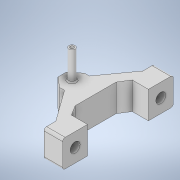
# Autodesk Inventor part: Base 2 LMU8
Saved by Autodesk Inventor 2022 (Build 260153000, 153)
## iProperties
Created: 2022-02-16
Part Number: Base 2 LMU8
Material: Genérico
Document SubType Name: Modeling
Designer: mathe
Density: 1 g/cm^3
Appearance: Padrão
Author: mathe
## iProperties of the stored document Base 2 LMU8_3DPrint.ipt
Created: 2022-02-18
Part Number: Base 2 LMU8_3DPrint
Material: Genérico
Document SubType Name: Modeling
Designer: mathe
Density: 1 g/cm^3
Appearance: Padrão
Author: mathe
Autodesk Inventor part; units mm, degrees
ref_plane "YZ Plane" through (0, 0, 0) normal (1, 0, 0) x (0, 1, 0)
ref_plane "XZ Plane" through (0, 0, 0) normal (0, 1, 0) x (-1, 0, 0)
ref_plane "XY Plane" through (0, 0, 0) normal (0, 0, 1) x (1, 0, 0)
sketch "Esboço1" plane through (0, 0, 0) normal (0, 1, 0) x (-1, 0, 0)
  line L0 (0, 0) -> (22, 0)
  line L1 (22, 0) -> (22, -22)
  line L2 (22, -22) -> (0, -22)
  line L3 (0, -22) -> (0, 0)
  dimension "d0" = 22
  dimension "d1" = 22
  constraints: 8 end point, 2 parallel, 1 horizontal, 1 perpendicular
  measures "d0" distance of L1.end L2.end
  measures "d1" distance of L0.end L1.end
extrude "Extrusão1" add sketch "Esboço1" along normal blind 20
sketch "Esboço2" plane through (0, 20, 0) normal (0, 1, 0) x (1, 0, 0)
  point P0 (0, 0)
  point P1 (-11, 11)
hole "Furo1" at (-11, 20, -11) direction (0, -1, 0) diameter 15 end through all
sketch "Esboço3" plane through (-22, 0, -22) normal (-1, 0, 0) x (0, 0, 1)
  line L0 (22, 0) -> (22, 20) projected
  line L1 (22, 10) -> (22, -34.5)
  line L2 (22, 10) -> (22, 54.5)
  line L3 (22, -34.5) -> (37, -34.5)
  line L4 (37, -34.5) -> (37, 54.5)
  line L5 (37, 54.5) -> (22, 54.5)
  line L6 (22, 54.5) -> (22, -34.5)
  dimension "d13" = 15
  constraints: 12 end point, 2 parallel, 1 collinear, 1 horizontal, 1 midpoint, 1 perpendicular, 1 point on line
  measures "d13" distance of L5.end L4.end
extrude "Extrusão2" add sketch "Esboço3" against normal up to surface (22 mm away)
chamfer "Chanfro1" distance 18 distance2 25 1 edges at (-11, 0, 0) measured on face at (-11, 0, -0.5)
sketch "Esboço4" plane through (-22, -34.5, 15) normal (0, 0, 1) x (1, 0, 0)
  line L0 (0, 89) -> (22, 89) projected
  point P0 (22, 34.5)
  point P1 (11, 10)
  point P2 (11, 79)
  dimension "d20" = 10
  measures "d20" distance from line of L0 point (11, 79)
hole "Furo2" at (-11, -24.5, 15) at (-11, 44.5, 15) direction (0, 0, -1) diameter 8 end through all
chamfer "Chanfro3" distance 18 distance2 25 1 edges at (-11, 20, 0) measured on face at (-11, 20, -0.5)
fillet "Arredondamento2" radius 2 4 edges at (0, 54.5, 7.5) (-22, 54.5, 7.5) (0, -34.5, 7.5) (-22, -34.5, 7.5)
sketch "Esboço10" plane through (-22, -32.5, 15) normal (0, 0, 1) x (1, 0, 0)
  line L0 (22, 77.5) -> (22, 52.5) projected
  line L1 (0, 7.5) -> (0, 32.5) projected
  line L2 (22, 67) -> (0, 67)
  line L3 (0, 67) -> (0, 18)
  line L4 (0, 18) -> (22, 18)
  line L5 (22, 18) -> (22, 67)
  circle A0 centre (11, 77) radius 4 projected
  circle A1 centre (11, 8) radius 4 projected
  point P0 (22, 32.5)
  dimension "d68" = 10
  dimension "d70" = 10
  constraints: 8 end point, 2 parallel, 2 point on line, 1 horizontal, 1 perpendicular
  measures "d68" distance from line of A0.centre L2
  measures "d70" distance from line of L4 A1.centre
extrude "Extrusão5" cut sketch "Esboço10" against normal blind 18 contours L0 L5 L4 L1 L3 L2
chamfer "Chanfro6" distance 5 distance2 8 1 edges at (-11, -14.5, -3) measured on face at (-11, -14.5, -2.5)
chamfer "Chanfro7" distance 5 distance2 8 1 edges at (-11, 34.5, -3) measured on face at (-11, 34.5, -2.5)
sketch "Esboço12" plane through (-22, 0, -22) normal (-1, 0, 0) x (0, 0, 1)
  line L0 (0, 0) -> (0, 20) projected
  arc A0 (0, 13) -> (0, 7) centre (0, 10) ccw
  line L1 (0, 0) -> (-8, 0)
  line L2 (-8, 0) -> (-8, 20)
  line L3 (-8, 20) -> (0, 20)
  line L4 (0, 20) -> (0, 0)
  line L5 (0, 0) -> (4, 0) projected
  line L6 (0, 0) -> (-8, 6.7128)
  line L7 (0, 0) -> (10.4433, 0) construction
  line L8 (0, 20) -> (-8, 13.2872)
  line L9 (0, 20) -> (10.4433, 20) construction
  circle A1 centre (0, 10) radius 3
  circle A2 centre (0, 10) radius 1.5
  point P0 (22, 0)
  point P1 (0, 11.5)
  point P2 (0, 8.5)
  point P3 (0, 13)
  point P4 (0, 13)
  dimension "d79" = 3
  dimension "d81" = 8
  dimension "d82" = 140
  dimension "d83" = 140
  dimension "d84" = 3
  constraints: 16 end point, 3 horizontal, 3 point on line, 2 centre point, 2 coincident, 2 equal length, 2 parallel, 2 point on circle, 1 midpoint, 1 perpendicular, 3 other
  measures "d79" radius of A0
  measures "d81" distance of L2.end L3.end
  measures "d82" angle of L7 L6
  measures "d83" angle of L8 L9
  measures "d84" diameter of A2
extrude "Extrusão6" cut sketch "Esboço12" against normal through all contours L0 A2 picked at (0.8735, 9.6865)
extrude "Extrusão7" add sketch "Esboço12" against normal up to surface (22 mm away) contours L6 L2 L8 L0 A0
extrude "Extrusão8" add sketch "Esboço12" against normal blind 21 contours A0 L0 A2
sketch "Esboço13" plane through (0, 45, 0) normal (1, 0, 0) x (0, 0, -1)
  circle A0 centre (22, -35) radius 1.5 projected
  circle A1 centre (22, -35) radius 1.5
  circle A2 centre (22, -35) radius 3
  circle A3 centre (22, -35) radius 2.5
  point P0 (0, -45)
  dimension "d99" = 5
  constraints: 3 centre point, 3 coincident
  measures "d99" diameter of A3
extrude "Extrusão11" add sketch "Esboço13" against normal blind 10 contours A2 | A3
extrude "Extrusão12" add sketch "Esboço13" along normal blind 23 contours A3
chamfer "Chanfro8" distance 1 angle 45 1 edges at (0, 10, -19.5)
